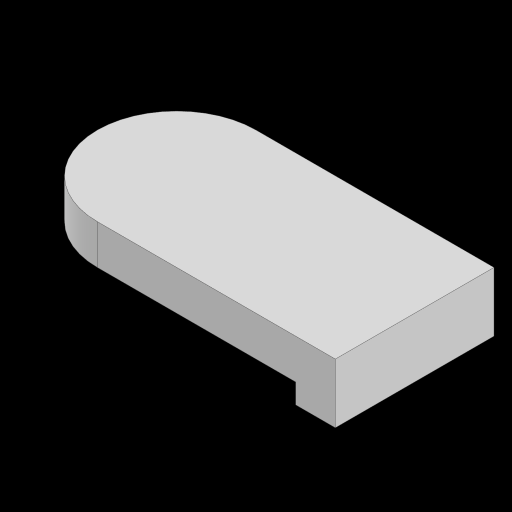
# Autodesk Inventor part: ANS9-3-BK
Saved by Autodesk Inventor 2024 (Build 280153000, 153)
## iProperties
Created: 2023-10-29
Part Number: ANS9-3-BK
Material: Generic
Document SubType Name: Modeling
Designer: bennk
Density: 1 g/cm^3
Appearance: Default
Author: bennk
Autodesk Inventor part; units mm, degrees
ref_plane "YZ Plane" through (0, 0, 0) normal (1, 0, 0) x (0, 1, 0)
ref_plane "XZ Plane" through (0, 0, 0) normal (0, 1, 0) x (-1, 0, 0)
ref_plane "XY Plane" through (0, 0, 0) normal (0, 0, 1) x (1, 0, 0)
sketch "Sketch1" plane through (0, 0, 0) normal (0, 1, 0) x (-1, 0, 0)
  circle A0 centre (0, 0) radius 25.4
  line L0 (0, 25.4) -> (-76.2, 25.4)
  line L1 (-76.2, 25.4) -> (-76.2, -25.4)
  line L2 (-76.2, -25.4) -> (0, -25.4)
  line L3 (0, -25.4) -> (0, 25.4)
  dimension "d0" = 50.8
  dimension "d1" = 76.2
  constraints: 8 end point, 2 parallel, 2 point on circle, 1 centre point, 1 coincident, 1 horizontal, 1 midpoint, 1 perpendicular
  measures "d0" diameter of A0
  measures "d1" distance of L2.end L1.end
extrude "Extrusion1" add sketch "Sketch1" against normal blind 12.7
sketch "Sketch2" plane through (76.2, 0, 25.4) normal (1, 0, 0) x (0, 0, -1)
  line L0 (50.8, -12.7) -> (0, -12.7) projected
  line L1 (0, -12.7) -> (50.8, -12.7)
  line L2 (50.8, -12.7) -> (50.8, -19.05)
  line L3 (50.8, -19.05) -> (0, -19.05)
  line L4 (0, -19.05) -> (0, -12.7)
  point P0 (25.4, 0)
  dimension "d4" = 6.35
  constraints: 8 end point, 2 parallel, 1 horizontal, 1 perpendicular, 1 point on line
  measures "d4" distance of L3.end L0.end
extrude "Extrusion2" add sketch "Sketch2" against normal blind 12.7
body "Solid1"
